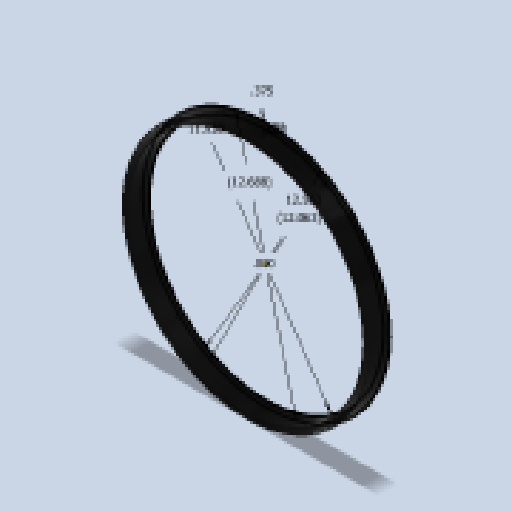
# Autodesk Inventor part: tubecap
Saved by Autodesk Inventor 2023 (Build 270158000, 158)
## iProperties
Created: 2022-10-12
Part Number: tubecap
Material: Generic
Document SubType Name: Modeling
Designer: Nathan
Density: 1 g/cm^3
Appearance: Glossy - Black
Mass: 89.1374 g
Surface Area: 1154.18 cm^2
Volume: 89.1374 cm^3
Author: Nathan
Autodesk Inventor part; units mm, degrees
ref_plane "YZ Plane" through (0, 0, 0) normal (1, 0, 0) x (0, 1, 0)
ref_plane "XZ Plane" through (0, 0, 0) normal (0, 1, 0) x (-1, 0, 0)
ref_plane "XY Plane" through (0, 0, 0) normal (0, 0, 1) x (1, 0, 0)
sketch "Sketch1" plane through (0, 0, 0) normal (0, 0, 1) x (1, 0, 0)
  circle A0 centre (0, 0) radius 161.1312
  circle A1 centre (0, 0) radius 151.6062
  circle A2 centre (0, 0) radius 153.1937
  circle A3 centre (0, 0) radius 159.5438
  dimension "d2" = 9.525
  dimension "d3" = 303.2125
  dimension "d4" = 322.2625
  dimension "d13" = 306.3875
  dimension "d14" = 319.0875
  dimension "d15" = 6.35
  dimension "d16" = 1.5875
  dimension "d21" = 0
  constraints: 4 centre point, 2 coincident
  measures "d2" radial gap between concentric circles of A1 A0
  measures "d3" diameter of A1
  measures "d4" diameter of A0
  measures "d13" diameter of A2
  measures "d14" diameter of A3
  measures "d15" radial gap between concentric circles of A2 A3
  measures "d16" radial gap between concentric circles of A3 A0
  measures "d21" distance of point (0, 0) A0.centre
extrude "Extrusion1" add sketch "Sketch1" along normal blind 1.5875 contours A3
extrude "Extrusion2" add sketch "Sketch1" along normal blind 25.4
body "Solid1"
